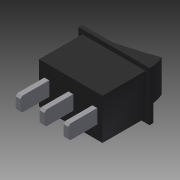
# Autodesk Inventor part: Toggle switch
Saved by Autodesk Inventor 2015 (Build 190159000, 159)
## iProperties
Created: 2016-10-18
Part Number: Toggle switch
Material: Generic
Document SubType Name: Modeling
Designer: James Yelland
Density: 1 g/cm^3
Appearance: Default
Author: James Yelland
Autodesk Inventor part; units mm, degrees
ref_plane "YZ Plane" through (0, 0, 0) normal (1, 0, 0) x (0, 1, 0)
ref_plane "XZ Plane" through (0, 0, 0) normal (0, 1, 0) x (-1, 0, 0)
ref_plane "XY Plane" through (0, 0, 0) normal (0, 0, 1) x (1, 0, 0)
sketch "Sketch1" plane through (0, 0, 0) normal (0, 1, 0) x (-1, 0, 0)
  line L0 (-6.6, 4.25) -> (-6.6, -4.25)
  line L1 (-6.6, -4.25) -> (6.6, -4.25)
  line L2 (6.6, -4.25) -> (6.6, 4.25)
  line L3 (6.6, 4.25) -> (-6.6, 4.25)
  line L4 (-6.6, 4.25) -> (6.6, -4.25) construction
  line L5 (-6.6, -4.25) -> (6.6, 4.25) construction
  point P0 (0, 0)
  dimension "d0" = 8.5
  dimension "d1" = 13.2
  constraints: 12 end point, 2 midpoint, 2 parallel, 1 perpendicular, 1 vertical
  measures "d0" distance of L0.start L0.end
  measures "d1" distance of L1.end L0.end
extrude "Extrusion1" add sketch "Sketch1" along normal blind 9
sketch "Sketch2" plane through (0, 9, 0) normal (0, 1, 0) x (1, 0, 0)
  line L0 (7.4, -5.15) -> (7.4, 5.15)
  line L1 (7.4, 5.15) -> (-7.4, 5.15)
  line L2 (-7.4, 5.15) -> (-7.4, -5.15)
  line L3 (-7.4, -5.15) -> (7.4, -5.15)
  line L4 (7.4, -5.15) -> (-7.4, 5.15) construction
  line L5 (7.4, 5.15) -> (-7.4, -5.15) construction
  point P0 (0, 0)
  dimension "d4" = 10.3
  dimension "d5" = 14.8
  constraints: 12 end point, 2 midpoint, 2 parallel, 1 perpendicular, 1 vertical
  measures "d4" distance of L0.start L0.end
  measures "d5" distance of L1.end L0.end
extrude "Extrusion2" add sketch "Sketch2" along normal blind 2
chamfer "Chamfer1" distance 1.8 distance2 1.2 1 edges at (7.4, 11, 0) measured on face at (6.9, 11, 0)
chamfer "Chamfer2" distance 1.8 distance2 1.2 1 edges at (-0.9, 11, 5.15) measured on face at (-0.9, 11, 4.65)
chamfer "Chamfer3" distance 1.8 distance2 1.2 1 edges at (-7.4, 11, -0.9) measured on face at (-6.9, 11, -0.9)
chamfer "Chamfer4" distance 1.8 distance2 1.2 1 edges at (0, 11, -5.15) measured on face at (0, 11, -4.65)
sketch "Sketch3" plane through (0, 11, 0) normal (0, 1, 0) x (1, 0, 0)
  line L0 (-5.6, 3.35) -> (5.6, 3.35) projected
  line L1 (-5.6, -3.35) -> (-5.6, 3.35) projected
  line L2 (5.6, -3.35) -> (-5.6, -3.35) projected
  line L3 (5.6, 3.35) -> (5.6, -3.35) projected
  point P0 (0, 0)
extrude "Extrusion3" add sketch "Sketch3" along normal blind 3
sketch "Sketch4" plane through (-5.6, 11, 3.35) normal (0, 0, 1) x (1, 0, 0)
  line L0 (11.2, 0) -> (0, 0) projected
  line L1 (11.2, 0) -> (11.2, 3) projected
  line L2 (0, 3) -> (11.2, 3) projected
  line L3 (0, 0) -> (0, 3) projected
  line L4 (11.2, 0) -> (11.2, 3)
  line L5 (11.2, 3) -> (0, 3)
  line L6 (0, 3) -> (0, 0)
  line L7 (0, 0) -> (11.2, 0)
  line L8 (11.2, 0) -> (10.5, 0)
  line L9 (11.2, 0) -> (0, 0) projected
  line L10 (10.5, 0) -> (10.5, 3)
  line L11 (0, 3) -> (11.2, 3) projected
  arc A0 (0, 0) -> (10.5, 3) centre (-15.0259, 72.4657) ccw
  arc A1 (11.2, 0) -> (10.5, 3) centre (4.6425, 0.0516) ccw
  point P0 (5.6, -11)
  dimension "d24" = 0.7
  constraints: 12 end point, 4 point on circle, 3 collinear, 2 centre point, 2 point on line, 1 perpendicular, 1 vertical
  measures "d24" distance of L7.end L8.end
extrude "Extrusion4" cut sketch "Sketch4" against normal through all contours A1 L2 L1 | A0 L3 L2
sketch "Sketch5" plane through (0, 0, 0) normal (0, -1, 0) x (1, 0, 0)
  line L0 (0.5, -1.5) -> (0.5, 1.5)
  line L1 (0.5, 1.5) -> (-0.5, 1.5)
  line L2 (-0.5, 1.5) -> (-0.5, -1.5)
  line L3 (-0.5, -1.5) -> (0.5, -1.5)
  line L4 (0.5, -1.5) -> (-0.5, 1.5) construction
  line L5 (0.5, 1.5) -> (-0.5, -1.5) construction
  line L6 (0, 0) -> (-5, 0)
  line L7 (0, 0) -> (5, 0)
  line L8 (-4.5, -1.5) -> (-4.5, 1.5)
  line L9 (-4.5, 1.5) -> (-5.5, 1.5)
  line L10 (-5.5, 1.5) -> (-5.5, -1.5)
  line L11 (-5.5, -1.5) -> (-4.5, -1.5)
  line L12 (-4.5, -1.5) -> (-5.5, 1.5) construction
  line L13 (-4.5, 1.5) -> (-5.5, -1.5) construction
  line L14 (5.5, -1.5) -> (5.5, 1.5)
  line L15 (5.5, 1.5) -> (4.5, 1.5)
  line L16 (4.5, 1.5) -> (4.5, -1.5)
  line L17 (4.5, -1.5) -> (5.5, -1.5)
  line L18 (5.5, -1.5) -> (4.5, 1.5) construction
  line L19 (5.5, 1.5) -> (4.5, -1.5) construction
  dimension "d27" = 3
  dimension "d28" = 1
  dimension "d29" = 5
  dimension "d30" = 5
  dimension "d31" = 1
  dimension "d32" = 1
  dimension "d41" = 3
  dimension "d42" = 3
  constraints: 40 end point, 6 midpoint, 6 parallel, 5 perpendicular, 2 vertical, 1 horizontal
  measures "d27" distance of L0.start L0.end
  measures "d28" distance of L1.end L0.end
  measures "d29" distance of L6.start L6.end
  measures "d30" distance of L6.start L7.end
  measures "d31" distance of L9.end L8.end
  measures "d32" distance of L15.end L14.end
  measures "d41" distance of L15.end L16.end
  measures "d42" distance of L8.start L8.end
extrude "Extrusion5" add sketch "Sketch5" along normal blind 6
chamfer "Chamfer5" distance 0.4 angle 45 6 edges at (5, -6, -1.5) (5, -6, 1.5) (0, -6, 1.5) (-5, -6, 1.5) (-5, -6, -1.5) (0, -6, -1.5)
body "Solid1"
